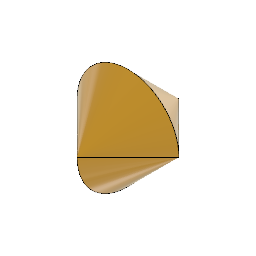
Sphericon (Autodesk Fusion 360 design; units mm, degrees)
Autodesk Fusion 360 part; units mm, degrees
sketch "Profile" plane through (0, 0, 0) normal (0, 0, 1) x (1, 0, 0)
  line L0 (50, 0) -> (0, 50)
  line L1 (0, 50) -> (-50, 0)
  line L2 (-50, 0) -> (0, -50)
  line L3 (0, -50) -> (50, 0)
  line L4 (-50, 0) -> (50, 0)
  dimension "d1" = 50
revolve "Revolve1" add sketch "Profile" angle 360 about axis through (-50, 0, 0) along (1, 0, 0) contours L0 L1 L4 makes body 1
split "Split1" by plane through (0, 0, 0) normal (0, 0, 1) bodies 1 makes body 2 at (-8.3333, 37.7828, 17.5663)
move_body "Move1" bodies 2 to x (0, -1, 0) y (1, 0, 0) z (0, 0, 1) at (0, 0, 0)
sketch "Holes" plane through (0, 0, 0) normal (0, 0, 1) x (1, 0, 0)
  circle A0 centre (-10, -17.3205) radius 2.6
  circle A1 centre (20, 0) radius 2.6
  circle A2 centre (0, 0) radius 5
  circle A3 centre (-20, 0) radius 2.6
  circle A4 centre (10, -17.3205) radius 2.6
  circle A5 centre (-10, 17.3205) radius 2.6
  circle A6 centre (0, 0) radius 20 construction
  circle A7 centre (10, 17.3205) radius 2.6
  dimension "d5" = 360
  dimension "d6" = 10
  dimension "d7" = 40
  dimension "d8" = 5.2
  measures "d6" diameter of A2
  measures "d7" diameter of A6
  measures "d8" diameter of A1
extrude "Extrude1" cut sketch "Holes" along normal mid plane 32 contours A2 bodies 1 2
extrude "Extrude2" cut sketch "Holes" along normal mid plane 14 contours A0 | A1 | A3 | A4 | A5 | A7 bodies 1 2
chamfer "Chamfer1" distance 5 angle 45 1 edges at (-4.6616, -1.8081, 16) on bodies 2
chamfer "Chamfer2" distance 2.5 angle 45 6 edges at (7.5759, -18.2607, 7) (17.5759, -0.9402, 7) (7.5759, 16.3803, 7) (-12.4241, 16.3803, 7) (-22.4241, -0.9402, 7) (-12.4241, -18.2607, 7) on bodies 2
named bodies: "Bottom", "Top"
